Autodesk Inventor part; units mm, degrees
(part 2 of 2)
sketch "ShorterHoneycomb" plane through (90.8296, 0, 51.7191) normal (1, 0, 0) x (0, 0, -1)
  line L0 (0, 131) -> (118, 131)
  line L1 (118, 131) -> (118, 0)
  line L2 (118, 0) -> (0, 0)
  line L3 (0, 0) -> (0, 131)
  line L4 (4, 131) -> (114, 131)
  line L5 (114, 131) -> (114, 0)
  line L6 (114, 0) -> (4, 0)
  line L7 (4, 0) -> (4, 131)
  line L8 (16.3923, 116) -> (9.4641, 116)
  line L9 (9.4641, 116) -> (6, 122)
  line L10 (6, 122) -> (9.4641, 128)
  line L11 (9.4641, 128) -> (16.3923, 128)
  line L12 (16.3923, 128) -> (19.8564, 122)
  line L13 (19.8564, 122) -> (16.3923, 116)
  line L14 (27.9393, 108) -> (21.0111, 108)
  line L15 (21.0111, 108) -> (17.547, 114)
  line L16 (17.547, 114) -> (21.0111, 120)
  line L17 (21.0111, 120) -> (27.9393, 120)
  line L18 (27.9393, 120) -> (31.4034, 114)
  line L19 (31.4034, 114) -> (27.9393, 108)
  line L20 (0, 131) -> (118, 131) projected
  line L21 (19.8564, 122) -> (21.0111, 120) construction
  line L22 (16.3923, 116) -> (17.547, 114) construction
  line L23 (16.3923, 101) -> (9.4641, 101)
  line L24 (9.4641, 101) -> (6, 107)
  line L25 (6, 107) -> (9.4641, 113)
  line L26 (9.4641, 113) -> (16.3923, 113)
  line L27 (16.3923, 113) -> (19.8564, 107)
  line L28 (19.8564, 107) -> (16.3923, 101)
  line L29 (27.9393, 93) -> (21.0111, 93)
  line L30 (21.0111, 93) -> (17.547, 99)
  line L31 (17.547, 99) -> (21.0111, 105)
  line L32 (21.0111, 105) -> (27.9393, 105)
  line L33 (27.9393, 105) -> (31.4034, 99)
  line L34 (31.4034, 99) -> (27.9393, 93)
  line L35 (19.8564, 107) -> (21.0111, 105) construction
  line L36 (16.3923, 101) -> (17.547, 99) construction
  line L37 (16.3923, 86) -> (9.4641, 86)
  line L38 (9.4641, 86) -> (6, 92)
  line L39 (6, 92) -> (9.4641, 98)
  line L40 (9.4641, 98) -> (16.3923, 98)
  line L41 (16.3923, 98) -> (19.8564, 92)
  line L42 (19.8564, 92) -> (16.3923, 86)
  line L43 (27.9393, 78) -> (21.0111, 78)
  line L44 (21.0111, 78) -> (17.547, 84)
  line L45 (17.547, 84) -> (21.0111, 90)
  line L46 (21.0111, 90) -> (27.9393, 90)
  line L47 (27.9393, 90) -> (31.4034, 84)
  line L48 (31.4034, 84) -> (27.9393, 78)
  line L49 (19.8564, 92) -> (21.0111, 90) construction
  line L50 (16.3923, 86) -> (17.547, 84) construction
  line L51 (16.3923, 71) -> (9.4641, 71)
  line L52 (9.4641, 71) -> (6, 77)
  line L53 (6, 77) -> (9.4641, 83)
  line L54 (9.4641, 83) -> (16.3923, 83)
  line L55 (16.3923, 83) -> (19.8564, 77)
  line L56 (19.8564, 77) -> (16.3923, 71)
  line L57 (27.9393, 63) -> (21.0111, 63)
  line L58 (21.0111, 63) -> (17.547, 69)
  line L59 (17.547, 69) -> (21.0111, 75)
  line L60 (21.0111, 75) -> (27.9393, 75)
  line L61 (27.9393, 75) -> (31.4034, 69)
  line L62 (31.4034, 69) -> (27.9393, 63)
  line L63 (19.8564, 77) -> (21.0111, 75) construction
  line L64 (16.3923, 71) -> (17.547, 69) construction
  line L65 (16.3923, 56) -> (9.4641, 56)
  line L66 (9.4641, 56) -> (6, 62)
  line L67 (6, 62) -> (9.4641, 68)
  line L68 (9.4641, 68) -> (16.3923, 68)
  line L69 (16.3923, 68) -> (19.8564, 62)
  line L70 (19.8564, 62) -> (16.3923, 56)
  line L71 (27.9393, 48) -> (21.0111, 48)
  line L72 (21.0111, 48) -> (17.547, 54)
  line L73 (17.547, 54) -> (21.0111, 60)
  line L74 (21.0111, 60) -> (27.9393, 60)
  line L75 (27.9393, 60) -> (31.4034, 54)
  line L76 (31.4034, 54) -> (27.9393, 48)
  line L77 (19.8564, 62) -> (21.0111, 60) construction
  line L78 (16.3923, 56) -> (17.547, 54) construction
  line L79 (16.3923, 41) -> (9.4641, 41)
  line L80 (9.4641, 41) -> (6, 47)
  line L81 (6, 47) -> (9.4641, 53)
  line L82 (9.4641, 53) -> (16.3923, 53)
  line L83 (16.3923, 53) -> (19.8564, 47)
  line L84 (19.8564, 47) -> (16.3923, 41)
  line L85 (27.9393, 33) -> (21.0111, 33)
  line L86 (21.0111, 33) -> (17.547, 39)
  line L87 (17.547, 39) -> (21.0111, 45)
  line L88 (21.0111, 45) -> (27.9393, 45)
  line L89 (27.9393, 45) -> (31.4034, 39)
  line L90 (31.4034, 39) -> (27.9393, 33)
  line L91 (19.8564, 47) -> (21.0111, 45) construction
  line L92 (16.3923, 41) -> (17.547, 39) construction
  line L93 (16.3923, 26) -> (9.4641, 26)
  line L94 (9.4641, 26) -> (6, 32)
  line L95 (6, 32) -> (9.4641, 38)
  line L96 (9.4641, 38) -> (16.3923, 38)
  line L97 (16.3923, 38) -> (19.8564, 32)
  line L98 (19.8564, 32) -> (16.3923, 26)
  line L99 (27.9393, 18) -> (21.0111, 18)
  line L100 (21.0111, 18) -> (17.547, 24)
  line L101 (17.547, 24) -> (21.0111, 30)
  line L102 (21.0111, 30) -> (27.9393, 30)
  line L103 (27.9393, 30) -> (31.4034, 24)
  line L104 (31.4034, 24) -> (27.9393, 18)
  line L105 (19.8564, 32) -> (21.0111, 30) construction
  line L106 (16.3923, 26) -> (17.547, 24) construction
  line L107 (16.3923, 11) -> (9.4641, 11)
  line L108 (9.4641, 11) -> (6, 17)
  line L109 (6, 17) -> (9.4641, 23)
  line L110 (9.4641, 23) -> (16.3923, 23)
  line L111 (16.3923, 23) -> (19.8564, 17)
  line L112 (19.8564, 17) -> (16.3923, 11)
  line L113 (27.9393, 3) -> (21.0111, 3)
  line L114 (21.0111, 3) -> (17.547, 9)
  line L115 (17.547, 9) -> (21.0111, 15)
  line L116 (21.0111, 15) -> (27.9393, 15)
  line L117 (27.9393, 15) -> (31.4034, 9)
  line L118 (31.4034, 9) -> (27.9393, 3)
  line L119 (19.8564, 17) -> (21.0111, 15) construction
  line L120 (16.3923, 11) -> (17.547, 9) construction
  line L121 (39.4923, 116) -> (32.5641, 116)
  line L122 (32.5641, 116) -> (29.1, 122)
  line L123 (29.1, 122) -> (32.5641, 128)
  line L124 (32.5641, 128) -> (39.4923, 128)
  line L125 (39.4923, 128) -> (42.9564, 122)
  line L126 (42.9564, 122) -> (39.4923, 116)
  line L127 (51.0393, 108) -> (44.1111, 108)
  line L128 (44.1111, 108) -> (40.647, 114)
  line L129 (40.647, 114) -> (44.1111, 120)
  line L130 (44.1111, 120) -> (51.0393, 120)
  line L131 (51.0393, 120) -> (54.5034, 114)
  line L132 (54.5034, 114) -> (51.0393, 108)
  line L133 (42.9564, 122) -> (44.1111, 120) construction
  line L134 (39.4923, 116) -> (40.647, 114) construction
  line L135 (39.4923, 101) -> (32.5641, 101)
  line L136 (32.5641, 101) -> (29.1, 107)
  line L137 (29.1, 107) -> (32.5641, 113)
  line L138 (32.5641, 113) -> (39.4923, 113)
  line L139 (39.4923, 113) -> (42.9564, 107)
  line L140 (42.9564, 107) -> (39.4923, 101)
  line L141 (51.0393, 93) -> (44.1111, 93)
  line L142 (44.1111, 93) -> (40.647, 99)
  line L143 (40.647, 99) -> (44.1111, 105)
  line L144 (44.1111, 105) -> (51.0393, 105)
  line L145 (51.0393, 105) -> (54.5034, 99)
  line L146 (54.5034, 99) -> (51.0393, 93)
  line L147 (42.9564, 107) -> (44.1111, 105) construction
  line L148 (39.4923, 101) -> (40.647, 99) construction
  line L149 (39.4923, 86) -> (32.5641, 86)
  line L150 (32.5641, 86) -> (29.1, 92)
  line L151 (29.1, 92) -> (32.5641, 98)
  line L152 (32.5641, 98) -> (39.4923, 98)
  line L153 (39.4923, 98) -> (42.9564, 92)
  line L154 (42.9564, 92) -> (39.4923, 86)
  line L155 (51.0393, 78) -> (44.1111, 78)
  line L156 (44.1111, 78) -> (40.647, 84)
  line L157 (40.647, 84) -> (44.1111, 90)
  line L158 (44.1111, 90) -> (51.0393, 90)
  line L159 (51.0393, 90) -> (54.5034, 84)
  line L160 (54.5034, 84) -> (51.0393, 78)
  line L161 (42.9564, 92) -> (44.1111, 90) construction
  line L162 (39.4923, 86) -> (40.647, 84) construction
  line L163 (39.4923, 71) -> (32.5641, 71)
  line L164 (32.5641, 71) -> (29.1, 77)
  line L165 (29.1, 77) -> (32.5641, 83)
  line L166 (32.5641, 83) -> (39.4923, 83)
  line L167 (39.4923, 83) -> (42.9564, 77)
  line L168 (42.9564, 77) -> (39.4923, 71)
  line L169 (51.0393, 63) -> (44.1111, 63)
  line L170 (44.1111, 63) -> (40.647, 69)
  line L171 (40.647, 69) -> (44.1111, 75)
  line L172 (44.1111, 75) -> (51.0393, 75)
  line L173 (51.0393, 75) -> (54.5034, 69)
  line L174 (54.5034, 69) -> (51.0393, 63)
  line L175 (42.9564, 77) -> (44.1111, 75) construction
  line L176 (39.4923, 71) -> (40.647, 69) construction
  line L177 (39.4923, 56) -> (32.5641, 56)
  line L178 (32.5641, 56) -> (29.1, 62)
  line L179 (29.1, 62) -> (32.5641, 68)
  line L180 (32.5641, 68) -> (39.4923, 68)
  line L181 (39.4923, 68) -> (42.9564, 62)
  line L182 (42.9564, 62) -> (39.4923, 56)
  line L183 (51.0393, 48) -> (44.1111, 48)
  line L184 (44.1111, 48) -> (40.647, 54)
  line L185 (40.647, 54) -> (44.1111, 60)
  line L186 (44.1111, 60) -> (51.0393, 60)
  line L187 (51.0393, 60) -> (54.5034, 54)
  line L188 (54.5034, 54) -> (51.0393, 48)
  line L189 (42.9564, 62) -> (44.1111, 60) construction
  line L190 (39.4923, 56) -> (40.647, 54) construction
  line L191 (39.4923, 41) -> (32.5641, 41)
  line L192 (32.5641, 41) -> (29.1, 47)
  line L193 (29.1, 47) -> (32.5641, 53)
  line L194 (32.5641, 53) -> (39.4923, 53)
  line L195 (39.4923, 53) -> (42.9564, 47)
  line L196 (42.9564, 47) -> (39.4923, 41)
  line L197 (51.0393, 33) -> (44.1111, 33)
  line L198 (44.1111, 33) -> (40.647, 39)
  line L199 (40.647, 39) -> (44.1111, 45)
  line L200 (44.1111, 45) -> (51.0393, 45)
  line L201 (51.0393, 45) -> (54.5034, 39)
  line L202 (54.5034, 39) -> (51.0393, 33)
  line L203 (42.9564, 47) -> (44.1111, 45) construction
  line L204 (39.4923, 41) -> (40.647, 39) construction
  line L205 (39.4923, 26) -> (32.5641, 26)
  line L206 (32.5641, 26) -> (29.1, 32)
  line L207 (29.1, 32) -> (32.5641, 38)
  line L208 (32.5641, 38) -> (39.4923, 38)
  line L209 (39.4923, 38) -> (42.9564, 32)
  line L210 (42.9564, 32) -> (39.4923, 26)
  line L211 (51.0393, 18) -> (44.1111, 18)
  line L212 (44.1111, 18) -> (40.647, 24)
  line L213 (40.647, 24) -> (44.1111, 30)
  line L214 (44.1111, 30) -> (51.0393, 30)
  line L215 (51.0393, 30) -> (54.5034, 24)
  line L216 (54.5034, 24) -> (51.0393, 18)
  line L217 (42.9564, 32) -> (44.1111, 30) construction
  line L218 (39.4923, 26) -> (40.647, 24) construction
  line L219 (39.4923, 11) -> (32.5641, 11)
  line L220 (32.5641, 11) -> (29.1, 17)
  line L221 (29.1, 17) -> (32.5641, 23)
  line L222 (32.5641, 23) -> (39.4923, 23)
  line L223 (39.4923, 23) -> (42.9564, 17)
  line L224 (42.9564, 17) -> (39.4923, 11)
  line L225 (51.0393, 3) -> (44.1111, 3)
  line L226 (44.1111, 3) -> (40.647, 9)
  line L227 (40.647, 9) -> (44.1111, 15)
  line L228 (44.1111, 15) -> (51.0393, 15)
  line L229 (51.0393, 15) -> (54.5034, 9)
  line L230 (54.5034, 9) -> (51.0393, 3)
  line L231 (42.9564, 17) -> (44.1111, 15) construction
  line L232 (39.4923, 11) -> (40.647, 9) construction
  line L233 (62.5923, 116) -> (55.6641, 116)
  line L234 (55.6641, 116) -> (52.2, 122)
  line L235 (52.2, 122) -> (55.6641, 128)
  line L236 (55.6641, 128) -> (62.5923, 128)
  line L237 (62.5923, 128) -> (66.0564, 122)
  line L238 (66.0564, 122) -> (62.5923, 116)
  line L239 (74.1393, 108) -> (67.2111, 108)
  line L240 (67.2111, 108) -> (63.747, 114)
  line L241 (63.747, 114) -> (67.2111, 120)
  line L242 (67.2111, 120) -> (74.1393, 120)
  line L243 (74.1393, 120) -> (77.6034, 114)
  line L244 (77.6034, 114) -> (74.1393, 108)
  line L245 (66.0564, 122) -> (67.2111, 120) construction
  line L246 (62.5923, 116) -> (63.747, 114) construction
  line L247 (62.5923, 101) -> (55.6641, 101)
  line L248 (55.6641, 101) -> (52.2, 107)
  line L249 (52.2, 107) -> (55.6641, 113)
  line L250 (55.6641, 113) -> (62.5923, 113)
  line L251 (62.5923, 113) -> (66.0564, 107)
  line L252 (66.0564, 107) -> (62.5923, 101)
  line L253 (74.1393, 93) -> (67.2111, 93)
  line L254 (67.2111, 93) -> (63.747, 99)
  line L255 (63.747, 99) -> (67.2111, 105)
  line L256 (67.2111, 105) -> (74.1393, 105)
  line L257 (74.1393, 105) -> (77.6034, 99)
  line L258 (77.6034, 99) -> (74.1393, 93)
  line L259 (66.0564, 107) -> (67.2111, 105) construction
  line L260 (62.5923, 101) -> (63.747, 99) construction
  line L261 (62.5923, 86) -> (55.6641, 86)
  line L262 (55.6641, 86) -> (52.2, 92)
  line L263 (52.2, 92) -> (55.6641, 98)
  line L264 (55.6641, 98) -> (62.5923, 98)
  line L265 (62.5923, 98) -> (66.0564, 92)
  line L266 (66.0564, 92) -> (62.5923, 86)
  line L267 (74.1393, 78) -> (67.2111, 78)
  line L268 (67.2111, 78) -> (63.747, 84)
  line L269 (63.747, 84) -> (67.2111, 90)
  line L270 (67.2111, 90) -> (74.1393, 90)
  line L271 (74.1393, 90) -> (77.6034, 84)
  line L272 (77.6034, 84) -> (74.1393, 78)
  line L273 (66.0564, 92) -> (67.2111, 90) construction
  line L274 (62.5923, 86) -> (63.747, 84) construction
  line L275 (62.5923, 71) -> (55.6641, 71)
  line L276 (55.6641, 71) -> (52.2, 77)
  line L277 (52.2, 77) -> (55.6641, 83)
  line L278 (55.6641, 83) -> (62.5923, 83)
  line L279 (62.5923, 83) -> (66.0564, 77)
  line L280 (66.0564, 77) -> (62.5923, 71)
  line L281 (74.1393, 63) -> (67.2111, 63)
  line L282 (67.2111, 63) -> (63.747, 69)
  line L283 (63.747, 69) -> (67.2111, 75)
  line L284 (67.2111, 75) -> (74.1393, 75)
  line L285 (74.1393, 75) -> (77.6034, 69)
  line L286 (77.6034, 69) -> (74.1393, 63)
  line L287 (66.0564, 77) -> (67.2111, 75) construction
  line L288 (62.5923, 71) -> (63.747, 69) construction
  line L289 (62.5923, 56) -> (55.6641, 56)
  line L290 (55.6641, 56) -> (52.2, 62)
  line L291 (52.2, 62) -> (55.6641, 68)
  line L292 (55.6641, 68) -> (62.5923, 68)
  line L293 (62.5923, 68) -> (66.0564, 62)
  line L294 (66.0564, 62) -> (62.5923, 56)
  line L295 (74.1393, 48) -> (67.2111, 48)
  line L296 (67.2111, 48) -> (63.747, 54)
  line L297 (63.747, 54) -> (67.2111, 60)
  line L298 (67.2111, 60) -> (74.1393, 60)
  line L299 (74.1393, 60) -> (77.6034, 54)
  line L300 (77.6034, 54) -> (74.1393, 48)
  line L301 (66.0564, 62) -> (67.2111, 60) construction
  line L302 (62.5923, 56) -> (63.747, 54) construction
  line L303 (62.5923, 41) -> (55.6641, 41)
  line L304 (55.6641, 41) -> (52.2, 47)
  line L305 (52.2, 47) -> (55.6641, 53)
  line L306 (55.6641, 53) -> (62.5923, 53)
  line L307 (62.5923, 53) -> (66.0564, 47)
  line L308 (66.0564, 47) -> (62.5923, 41)
  line L309 (74.1393, 33) -> (67.2111, 33)
  line L310 (67.2111, 33) -> (63.747, 39)
  line L311 (63.747, 39) -> (67.2111, 45)
  line L312 (67.2111, 45) -> (74.1393, 45)
  line L313 (74.1393, 45) -> (77.6034, 39)
  line L314 (77.6034, 39) -> (74.1393, 33)
  line L315 (66.0564, 47) -> (67.2111, 45) construction
  line L316 (62.5923, 41) -> (63.747, 39) construction
  line L317 (62.5923, 26) -> (55.6641, 26)
  line L318 (55.6641, 26) -> (52.2, 32)
  line L319 (52.2, 32) -> (55.6641, 38)
  line L320 (55.6641, 38) -> (62.5923, 38)
  line L321 (62.5923, 38) -> (66.0564, 32)
  line L322 (66.0564, 32) -> (62.5923, 26)
  line L323 (74.1393, 18) -> (67.2111, 18)
  line L324 (67.2111, 18) -> (63.747, 24)
  line L325 (63.747, 24) -> (67.2111, 30)
  line L326 (67.2111, 30) -> (74.1393, 30)
  line L327 (74.1393, 30) -> (77.6034, 24)
  line L328 (77.6034, 24) -> (74.1393, 18)
  line L329 (66.0564, 32) -> (67.2111, 30) construction
  line L330 (62.5923, 26) -> (63.747, 24) construction
  line L331 (62.5923, 11) -> (55.6641, 11)
  line L332 (55.6641, 11) -> (52.2, 17)
  line L333 (52.2, 17) -> (55.6641, 23)
  line L334 (55.6641, 23) -> (62.5923, 23)
  line L335 (62.5923, 23) -> (66.0564, 17)
  line L336 (66.0564, 17) -> (62.5923, 11)
  line L337 (74.1393, 3) -> (67.2111, 3)
  line L338 (67.2111, 3) -> (63.747, 9)
  line L339 (63.747, 9) -> (67.2111, 15)
  line L340 (67.2111, 15) -> (74.1393, 15)
  line L341 (74.1393, 15) -> (77.6034, 9)
  line L342 (77.6034, 9) -> (74.1393, 3)
  line L343 (66.0564, 17) -> (67.2111, 15) construction
  line L344 (62.5923, 11) -> (63.747, 9) construction
  line L345 (85.6923, 116) -> (78.7641, 116)
  line L346 (78.7641, 116) -> (75.3, 122)
  line L347 (75.3, 122) -> (78.7641, 128)
  line L348 (78.7641, 128) -> (85.6923, 128)
  line L349 (85.6923, 128) -> (89.1564, 122)
  line L350 (89.1564, 122) -> (85.6923, 116)
  line L351 (97.2393, 108) -> (90.3111, 108)
  line L352 (90.3111, 108) -> (86.847, 114)
  line L353 (86.847, 114) -> (90.3111, 120)
  line L354 (90.3111, 120) -> (97.2393, 120)
  line L355 (97.2393, 120) -> (100.7034, 114)
  line L356 (100.7034, 114) -> (97.2393, 108)
  line L357 (89.1564, 122) -> (90.3111, 120) construction
  line L358 (85.6923, 116) -> (86.847, 114) construction
  line L359 (85.6923, 101) -> (78.7641, 101)
  line L360 (78.7641, 101) -> (75.3, 107)
  line L361 (75.3, 107) -> (78.7641, 113)
  line L362 (78.7641, 113) -> (85.6923, 113)
  line L363 (85.6923, 113) -> (89.1564, 107)
  line L364 (89.1564, 107) -> (85.6923, 101)
  line L365 (97.2393, 93) -> (90.3111, 93)
  line L366 (90.3111, 93) -> (86.847, 99)
  line L367 (86.847, 99) -> (90.3111, 105)
  line L368 (90.3111, 105) -> (97.2393, 105)
  line L369 (97.2393, 105) -> (100.7034, 99)
  line L370 (100.7034, 99) -> (97.2393, 93)
  line L371 (89.1564, 107) -> (90.3111, 105) construction
  line L372 (85.6923, 101) -> (86.847, 99) construction
  line L373 (85.6923, 86) -> (78.7641, 86)
  line L374 (78.7641, 86) -> (75.3, 92)
  line L375 (75.3, 92) -> (78.7641, 98)
  line L376 (78.7641, 98) -> (85.6923, 98)
  line L377 (85.6923, 98) -> (89.1564, 92)
  line L378 (89.1564, 92) -> (85.6923, 86)
  line L379 (97.2393, 78) -> (90.3111, 78)
  line L380 (90.3111, 78) -> (86.847, 84)
  line L381 (86.847, 84) -> (90.3111, 90)
  line L382 (90.3111, 90) -> (97.2393, 90)
  line L383 (97.2393, 90) -> (100.7034, 84)
  line L384 (100.7034, 84) -> (97.2393, 78)
  line L385 (89.1564, 92) -> (90.3111, 90) construction
  line L386 (85.6923, 86) -> (86.847, 84) construction
  line L387 (85.6923, 71) -> (78.7641, 71)
  line L388 (78.7641, 71) -> (75.3, 77)
  line L389 (75.3, 77) -> (78.7641, 83)
  line L390 (78.7641, 83) -> (85.6923, 83)
  line L391 (85.6923, 83) -> (89.1564, 77)
  line L392 (89.1564, 77) -> (85.6923, 71)
  line L393 (97.2393, 63) -> (90.3111, 63)
  line L394 (90.3111, 63) -> (86.847, 69)
  line L395 (86.847, 69) -> (90.3111, 75)
  line L396 (90.3111, 75) -> (97.2393, 75)
  line L397 (97.2393, 75) -> (100.7034, 69)
  line L398 (100.7034, 69) -> (97.2393, 63)
  line L399 (89.1564, 77) -> (90.3111, 75) construction
  line L400 (85.6923, 71) -> (86.847, 69) construction
  line L401 (85.6923, 56) -> (78.7641, 56)
  line L402 (78.7641, 56) -> (75.3, 62)
  line L403 (75.3, 62) -> (78.7641, 68)
  line L404 (78.7641, 68) -> (85.6923, 68)
  line L405 (85.6923, 68) -> (89.1564, 62)
  line L406 (89.1564, 62) -> (85.6923, 56)
  line L407 (97.2393, 48) -> (90.3111, 48)
  line L408 (90.3111, 48) -> (86.847, 54)
  line L409 (86.847, 54) -> (90.3111, 60)
  line L410 (90.3111, 60) -> (97.2393, 60)
  line L411 (97.2393, 60) -> (100.7034, 54)
  line L412 (100.7034, 54) -> (97.2393, 48)
  line L413 (89.1564, 62) -> (90.3111, 60) construction
  line L414 (85.6923, 56) -> (86.847, 54) construction
  line L415 (85.6923, 41) -> (78.7641, 41)
  line L416 (78.7641, 41) -> (75.3, 47)
  line L417 (75.3, 47) -> (78.7641, 53)
  line L418 (78.7641, 53) -> (85.6923, 53)
  line L419 (85.6923, 53) -> (89.1564, 47)
  line L420 (89.1564, 47) -> (85.6923, 41)
  line L421 (97.2393, 33) -> (90.3111, 33)
  line L422 (90.3111, 33) -> (86.847, 39)
  line L423 (86.847, 39) -> (90.3111, 45)
  line L424 (90.3111, 45) -> (97.2393, 45)
  line L425 (97.2393, 45) -> (100.7034, 39)
  line L426 (100.7034, 39) -> (97.2393, 33)
  line L427 (89.1564, 47) -> (90.3111, 45) construction
  line L428 (85.6923, 41) -> (86.847, 39) construction
  line L429 (85.6923, 26) -> (78.7641, 26)
  line L430 (78.7641, 26) -> (75.3, 32)
  line L431 (75.3, 32) -> (78.7641, 38)
  line L432 (78.7641, 38) -> (85.6923, 38)
  line L433 (85.6923, 38) -> (89.1564, 32)
  line L434 (89.1564, 32) -> (85.6923, 26)
  line L435 (97.2393, 18) -> (90.3111, 18)
  line L436 (90.3111, 18) -> (86.847, 24)
  line L437 (86.847, 24) -> (90.3111, 30)
  line L438 (90.3111, 30) -> (97.2393, 30)
  line L439 (97.2393, 30) -> (100.7034, 24)
  line L440 (100.7034, 24) -> (97.2393, 18)
  line L441 (89.1564, 32) -> (90.3111, 30) construction
  line L442 (85.6923, 26) -> (86.847, 24) construction
  line L443 (85.6923, 11) -> (78.7641, 11)
  line L444 (78.7641, 11) -> (75.3, 17)
  line L445 (75.3, 17) -> (78.7641, 23)
  line L446 (78.7641, 23) -> (85.6923, 23)
  line L447 (85.6923, 23) -> (89.1564, 17)
  line L448 (89.1564, 17) -> (85.6923, 11)
  line L449 (97.2393, 3) -> (90.3111, 3)
  line L450 (90.3111, 3) -> (86.847, 9)
  line L451 (86.847, 9) -> (90.3111, 15)
  line L452 (90.3111, 15) -> (97.2393, 15)
  line L453 (97.2393, 15) -> (100.7034, 9)
  line L454 (100.7034, 9) -> (97.2393, 3)
  line L455 (89.1564, 17) -> (90.3111, 15) construction
  line L456 (85.6923, 11) -> (86.847, 9) construction
  line L457 (108.6923, 116) -> (101.7641, 116)
  line L458 (101.7641, 116) -> (98.3, 122)
  line L459 (101.7641, 128) -> (108.6923, 128)
  line L460 (108.6923, 128) -> (112.1564, 122)
  line L461 (112.1564, 122) -> (108.6923, 116)
  line L462 (98.3, 122) -> (101.7641, 128)
  line L463 (108.6923, 101) -> (101.7641, 101)
  line L464 (101.7641, 101) -> (98.3, 107)
  line L465 (101.7641, 113) -> (108.6923, 113)
  line L466 (108.6923, 113) -> (112.1564, 107)
  line L467 (112.1564, 107) -> (108.6923, 101)
  line L468 (98.3, 107) -> (101.7641, 113)
  line L469 (108.6923, 86) -> (101.7641, 86)
  line L470 (101.7641, 86) -> (98.3, 92)
  line L471 (101.7641, 98) -> (108.6923, 98)
  line L472 (108.6923, 98) -> (112.1564, 92)
  line L473 (112.1564, 92) -> (108.6923, 86)
  line L474 (98.3, 92) -> (101.7641, 98)
  line L475 (108.6923, 71) -> (101.7641, 71)
  line L476 (101.7641, 71) -> (98.3, 77)
  line L477 (101.7641, 83) -> (108.6923, 83)
  line L478 (108.6923, 83) -> (112.1564, 77)
  line L479 (112.1564, 77) -> (108.6923, 71)
  line L480 (98.3, 77) -> (101.7641, 83)
  line L481 (108.6923, 56) -> (101.7641, 56)
  line L482 (101.7641, 56) -> (98.3, 62)
  line L483 (101.7641, 68) -> (108.6923, 68)
  line L484 (108.6923, 68) -> (112.1564, 62)
  line L485 (112.1564, 62) -> (108.6923, 56)
  line L486 (98.3, 62) -> (101.7641, 68)
  line L487 (108.6923, 41) -> (101.7641, 41)
  line L488 (101.7641, 41) -> (98.3, 47)
  line L489 (101.7641, 53) -> (108.6923, 53)
  line L490 (108.6923, 53) -> (112.1564, 47)
  line L491 (112.1564, 47) -> (108.6923, 41)
  line L492 (98.3, 47) -> (101.7641, 53)
  line L493 (108.6923, 26) -> (101.7641, 26)
  line L494 (101.7641, 26) -> (98.3, 32)
  line L495 (101.7641, 38) -> (108.6923, 38)
  line L496 (108.6923, 38) -> (112.1564, 32)
  line L497 (112.1564, 32) -> (108.6923, 26)
  line L498 (98.3, 32) -> (101.7641, 38)
  line L499 (108.6923, 11) -> (101.7641, 11)
  line L500 (101.7641, 11) -> (98.3, 17)
  line L501 (101.7641, 23) -> (108.6923, 23)
  line L502 (108.6923, 23) -> (112.1564, 17)
  line L503 (112.1564, 17) -> (108.6923, 11)
  line L504 (98.3, 17) -> (101.7641, 23)
  point P0 (51.7191, 0)
  point P1 (12.9282, 122)
  point P2 (24.4752, 114)
  point P3 (12.9282, 107)
  point P4 (24.4752, 99)
  point P5 (12.9282, 92)
  point P6 (24.4752, 84)
  point P7 (12.9282, 77)
  point P8 (24.4752, 69)
  point P9 (12.9282, 62)
  point P10 (24.4752, 54)
  point P11 (12.9282, 47)
  point P12 (24.4752, 39)
  point P13 (12.9282, 32)
  point P14 (24.4752, 24)
  point P15 (12.9282, 17)
  point P16 (24.4752, 9)
  point P17 (36.0282, 122)
  point P18 (47.5752, 114)
  point P19 (36.0282, 107)
  point P20 (47.5752, 99)
  point P21 (36.0282, 92)
  point P22 (47.5752, 84)
  point P23 (36.0282, 77)
  point P24 (47.5752, 69)
  point P25 (36.0282, 62)
  point P26 (47.5752, 54)
  point P27 (36.0282, 47)
  point P28 (47.5752, 39)
  point P29 (36.0282, 32)
  point P30 (47.5752, 24)
  point P31 (36.0282, 17)
  point P32 (47.5752, 9)
  point P33 (59.1282, 122)
  point P34 (70.6752, 114)
  point P35 (59.1282, 107)
  point P36 (70.6752, 99)
  point P37 (59.1282, 92)
  point P38 (70.6752, 84)
  point P39 (59.1282, 77)
  point P40 (70.6752, 69)
  point P41 (59.1282, 62)
  point P42 (70.6752, 54)
  point P43 (59.1282, 47)
  point P44 (70.6752, 39)
  point P45 (59.1282, 32)
  point P46 (70.6752, 24)
  point P47 (59.1282, 17)
  point P48 (70.6752, 9)
  point P49 (82.2282, 122)
  point P50 (93.7752, 114)
  point P51 (82.2282, 107)
  point P52 (93.7752, 99)
  point P53 (82.2282, 92)
  point P54 (93.7752, 84)
  point P55 (82.2282, 77)
  point P56 (93.7752, 69)
  point P57 (82.2282, 62)
  point P58 (93.7752, 54)
  point P59 (82.2282, 47)
  point P60 (93.7752, 39)
  point P61 (82.2282, 32)
  point P62 (93.7752, 24)
  point P63 (82.2282, 17)
  point P64 (93.7752, 9)
  point P65 (105.2282, 122)
  dimension "d32" = 12
  dimension "d33" = 2
  dimension "d35" = 3
  dimension "d36" = 2
  dimension "d39" = 15
  dimension "d42" = 23.1
  dimension "d56" = 2
  dimension "d57" = 3
  dimension "d58" = 1.5
  dimension "d59" = 1.5052
  dimension "d62" = 23
  constraints: 1008 end point, 7 parallel, 4 horizontal, 2 collinear, 2 perpendicular, 1 vertical, 991 other
  measures "d32" distance between parallel lines of L8 L11
  measures "d33" distance between parallel lines of L16 L13
  measures "d35" distance between parallel lines of L4 L11
  measures "d36" distance from line of L7 L9.end
  measures "d39" distance of L14.end L29.end
  measures "d42" distance of L14.end L127.end
  measures "d56" distance between parallel lines of L381 L378
  measures "d57" distance between parallel lines of L376 L359
  measures "d58" distance between parallel lines of L366 L377
  measures "d59" distance between parallel lines of L258 L375
  measures "d62" distance of point (82.228, 122) point (105.228, 122)
extrude "HoneycombShortSide" cut sketch "ShorterHoneycomb" against normal blind 200 contours L8 L9 L10 L11 L12 L13 | L14 L15 L16 L17 L18 L19 | L23 L24 L25 L26 L27 L28 | L29 L30 L31 L32 L33 L34 | L37 L38 L39 L40 L41 L42 | L43 L44 L45 L46 L47 L48 | L51 L52 L53 L54 L55 L56 | L57 L58 L59 L60 L61 L62 | L65 L66 L67 L68 L69 L70 | L71 L72 L73 L74 L75 L76 | L79 L80 L81 L82 L83 L84 | L85 L86 L87 L88 L89 L90 | L93 L94 L95 L96 L97 L98 | L99 L100 L101 L102 L103 L104 | L107 L108 L109 L110 L111 L112 | L113 L114 L115 L116 L117 L118 | L121 L122 L123 L124 L125 L126 | L127 L128 L129 L130 L131 L132 | L135 L136 L137 L138 L139 L140 | L141 L142 L143 L144 L145 L146 | L149 L150 L151 L152 L153 L154 | L155 L156 L157 L158 L159 L160 | L163 L164 L165 L166 L167 L168 | L169 L170 L171 L172 L173 L174 | L177 L178 L179 L180 L181 L182 | L183 L184 L185 L186 L187 L188 | L191 L192 L193 L194 L195 L196 | L197 L198 L199 L200 L201 L202 | L205 L206 L207 L208 L209 L210 | L211 L212 L213 L214 L215 L216 | L219 L220 L221 L222 L223 L224 | L225 L226 L227 L228 L229 L230 | L233 L234 L235 L236 L237 L238 | L239 L240 L241 L242 L243 L244 | L247 L248 L249 L250 L251 L252 | L253 L254 L255 L256 L257 L258 | L261 L262 L263 L264 L265 L266 | L267 L268 L269 L270 L271 L272 | L275 L276 L277 L278 L279 L280 | L281 L282 L283 L284 L285 L286 | L289 L290 L291 L292 L293 L294 | L295 L296 L297 L298 L299 L300 | L303 L304 L305 L306 L307 L308 | L309 L310 L311 L312 L313 L314 | L317 L318 L319 L320 L321 L322 | L323 L324 L325 L326 L327 L328 | L331 L332 L333 L334 L335 L336 | L337 L338 L339 L340 L341 L342 | L345 L346 L347 L348 L349 L350 | L351 L352 L353 L354 L355 L356 | L359 L360 L361 L362 L363 L364 | L365 L366 L367 L368 L369 L370 | L373 L374 L375 L376 L377 L378 | L379 L380 L381 L382 L383 L384 | L387 L388 L389 L390 L391 L392 | L393 L394 L395 L396 L397 L398 | L401 L402 L403 L404 L405 L406 | L407 L408 L409 L410 L411 L412 | L415 L416 L417 L418 L419 L420 | L421 L422 L423 L424 L425 L426 | L429 L430 L431 L432 L433 L434 | L435 L436 L437 L438 L439 L440 | L443 L444 L445 L446 L447 L448 | L449 L450 L451 L452 L453 L454 | L457 L458 L462 L459 L460 L461 | L463 L464 L468 L465 L466 L467 | L469 L470 L474 L471 L472 L473 | L475 L476 L480 L477 L478 L479 | L481 L482 L486 L483 L484 L485 | L487 L488 L492 L489 L490 L491 | L493 L494 L498 L495 L496 L497 | L499 L500 L504 L501 L502 L503
extrude "SidePanels" add sketch "BasicBox" along normal blind 131 contours L0 L42 L22 L18 L43 L3 | L43 L18 L40 L3 | L0 L1 L2 L44 L27 L25 L16 L24 L23 L17 L22 L42 | L40 L18 L26 L19 L27 L44 L2 L3
sketch "DroneAttachmentSide1" plane through (-92.1704, 0, 51.7191) normal (0, 0, 1) x (1, 0, 0)
  circle A0 centre (51.5, 138) radius 3.5
  circle A1 centre (131.5, 138) radius 3.5
  line L0 (51.5, 138) -> (131.5, 138) construction
  line L1 (0, 131) -> (183, 131) projected
  line L2 (51.5, 138) -> (51.5, 131) construction
  line L3 (179, 131) -> (4, 131) projected
  line L4 (131.5, 138) -> (131.5, 131) construction
  line L5 (0, 131) -> (51.5, 138)
  line L6 (131.5, 138) -> (183, 131)
  arc A2 (61.5, 138) -> (41.5911, 136.6532) centre (51.5, 138) ccw
  line L7 (61.5, 138) -> (67.3737, 131)
  line L8 (61.5, 138) -> (70.6379, 138) construction
  line L9 (0, 131) -> (67.3737, 131)
  arc A3 (141.4089, 136.6532) -> (121.5, 138) centre (131.5, 138) ccw
  line L10 (121.5, 138) -> (113.1577, 131)
  line L11 (121.5, 138) -> (130.7015, 138) construction
  line L12 (113.1577, 131) -> (183, 131)
  line L13 (183, 131) -> (0, 131) projected
  line L14 (0, 0) -> (183, 0) projected
  point P0 (92.1704, 0)
  dimension "d72" = 7
  dimension "d73" = 80
  dimension "d74" = 7
  dimension "d75" = 10
  dimension "d76" = 50
  dimension "d77" = 140
  dimension "d133" = 138
  constraints: 22 end point, 6 point on line, 4 centre point, 4 collinear, 4 point on circle, 2 coincident, 2 equal length, 2 equal radius, 2 horizontal, 2 perpendicular, 1 parallel
  measures "d72" diameter of A0
  measures "d73" distance of L0.start L0.end
  measures "d74" distance of L2.end L0.start
  measures "d75" radius of A2
  measures "d76" angle of L7 L8
  measures "d77" angle of L10 L11
  measures "d133" distance from line of L14 A2.centre
extrude "DroneAttachment1" add sketch "DroneAttachmentSide1" against normal blind 4
sketch "Sketch5" plane through (90.8296, 0, -66.2809) normal (0, 0, -1) x (-1, 0, 0)
  circle A0 centre (51.5, 138) radius 3.5 projected
  circle A1 centre (51.5, 138) radius 3.5
  circle A2 centre (131.5, 138) radius 3.5 projected
  circle A3 centre (131.5, 138) radius 3.5
  line L0 (69.8423, 131) -> (0, 131)
  line L1 (0, 131) -> (41.5911, 136.6532)
  line L2 (0, 131) -> (41.5911, 136.6532) projected
  line L3 (69.8423, 131) -> (61.5, 138)
  line L4 (69.8423, 131) -> (61.5, 138) projected
  arc A4 (61.5, 138) -> (41.5911, 136.6532) centre (51.5, 138) ccw
  line L5 (121.5, 138) -> (115.6263, 131)
  line L6 (121.5, 138) -> (115.6263, 131) projected
  line L7 (115.6263, 131) -> (183, 131)
  line L8 (183, 131) -> (141.4089, 136.6532)
  line L9 (183, 131) -> (141.4089, 136.6532) projected
  arc A5 (141.4089, 136.6532) -> (121.5, 138) centre (131.5, 138) ccw
  point P0 (90.8296, 0)
  constraints: 12 end point, 4 centre point, 4 coincident, 4 collinear, 4 point on circle, 2 horizontal
extrude "Droneattachment2" add sketch "Sketch5" against normal blind 4
sketch "PowerButton" plane through (90.8296, 0, 51.7191) normal (1, 0, 0) x (0, 0, -1)
  line L0 (0, 131) -> (118, 131)
  line L1 (118, 131) -> (118, 0)
  line L2 (118, 0) -> (0, 0)
  line L3 (0, 0) -> (0, 131)
  line L4 (4, 131) -> (114, 131)
  line L5 (114, 131) -> (114, 0)
  line L6 (114, 0) -> (4, 0)
  line L7 (4, 0) -> (4, 131)
  circle A0 centre (24, 61) radius 9.5
  point P0 (51.7191, 0)
  dimension "d82" = 19
  dimension "d83" = 20
  dimension "d84" = 70
  constraints: 16 end point, 4 parallel, 2 horizontal, 2 perpendicular, 1 centre point
  measures "d82" diameter of A0
  measures "d83" distance from line of L7 A0.centre
  measures "d84" distance from line of L0 A0.centre
extrude "PowerButtonSupport" add sketch "PowerButton" against normal blind 7 contours A0
hole "PowerButtonHole" at (90.8296, 61, 27.7191) direction (-1, 0, 0) diameter 15.7 depth 20 tip angle 118
extrude "LensplateMount" add sketch "BasicBox" along normal blind 15 contours L3 L58 L0 | L58 L59 L60 L61 L62 L0 | L3 L39 L38 L0 L62 L61 L60 L59 | L40 L18 L26 L19 L27 L44 L2 L3 | L3 L64 L69 L68 L67 L2 L41 L40 | L36 L37 L1 L55 L54 L53 L52 L0 | L65 L2 L67 L68 L69 L64 | L3 L2 L65 | L45 L7 L6 L44 L27 L19 L26 L18 | L52 L53 L54 L55 L56 L0 | L56 L1 L0 | L2 L47 L46 L51 L50 L1 L35 L34 | L2 L49 L50 L51 L46 L47 | L49 L2 L1
extrude "LensplateaAttachment" add sketch "BasicBox" along normal blind 20 contours L3 L58 L0 | L3 L39 L38 L0 L62 L61 L60 L59 | L40 L18 L26 L19 L27 L44 L2 L3 | L3 L64 L69 L68 L67 L2 L41 L40 | L36 L37 L1 L55 L54 L53 L52 L0 | L3 L2 L65 | L45 L7 L6 L44 L27 L19 L26 L18 | L56 L1 L0 | L2 L47 L46 L51 L50 L1 L35 L34 | L49 L2 L1
sketch "stuffplate_Mount" plane through (-92.1704, 0, 51.7191) normal (0, 0, 1) x (1, 0, 0)
  line L0 (0, 131) -> (183, 131)
  line L1 (183, 131) -> (183, 0)
  line L2 (183, 0) -> (0, 0)
  line L3 (0, 0) -> (0, 131)
  line L4 (0, 106) -> (183, 106)
  line L5 (0, 98) -> (183, 98)
  circle A0 centre (75, 102) radius 3
  circle A1 centre (135, 102) radius 3
  line L6 (75, 102) -> (135, 102) construction
  line L7 (144.4393, 76) -> (137.5111, 76) projected
  line L8 (109.7923, 84) -> (102.8641, 84) projected
  line L9 (135, 102) -> (183, 102) construction
  line L10 (183, 84) -> (183, 78) projected
  line L11 (75, 102) -> (0, 102) construction
  line L12 (0, 77) -> (0, 83) projected
  line L13 (75, 102) -> (75, 98) construction
  line L14 (75, 102) -> (75, 106) construction
  line L15 (135, 102) -> (135, 106) construction
  line L16 (135, 102) -> (135, 98) construction
  point P0 (92.1704, 0)
  dimension "d111" = 8
  dimension "d112" = 6
  dimension "d116" = 48
  dimension "d117" = 60
  dimension "d118" = 75
  dimension "d119" = 25
  constraints: 26 end point, 12 point on line, 5 parallel, 5 perpendicular, 2 centre point, 2 equal length, 2 horizontal, 1 equal radius
  measures "d111" distance between parallel lines of L5 L4
  measures "d112" diameter of A0
  measures "d116" distance of L4.end L15.end
  measures "d117" distance of L14.end L15.end
  measures "d118" distance of L14.end L4.start
  measures "d119" distance between parallel lines of L0 L4
extrude "StuffplateMount" add sketch "stuffplate_Mount" against normal blind 6 contours L4 L1 L5 L3 | A0 | A1
sketch "Sketch8" plane through (90.8296, 0, -66.2809) normal (0, 0, -1) x (-1, 0, 0)
  line L0 (179, 106) -> (4, 106)
  line L1 (4, 106) -> (4, 98)
  line L2 (4, 98) -> (179, 98)
  line L3 (179, 98) -> (179, 106)
  point P0 (90.8296, 0)
  dimension "d122" = 8
  dimension "d123" = 175
  constraints: 8 end point, 2 parallel, 1 horizontal, 1 perpendicular
  measures "d122" distance between parallel lines of L2 L0
  measures "d123" distance between parallel lines of L3 L1
extrude "StuffplateMount2" add sketch "Sketch8" against normal blind 6
hole "Hole2" at (-92.1704, 131, 51.7191) at (90.8296, 0, 51.7191) at (-17.1704, 102, 51.7191) at (42.8296, 102, 51.7191) direction (0, 0, -1) diameter 2 end through all
body "Solid1"
